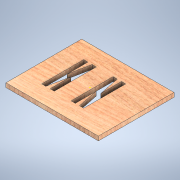
# Autodesk Inventor part: Parte A-B
Saved by Autodesk Inventor 2022 (Build 260153000, 153)
## iProperties
Created: 2023-02-12
Part Number: Parte A-B
Material: Madera (abedul)
Document SubType Name: Modeling
Designer: USUARIO
Density: 0.55 g/cm^3
Appearance: Abedul - Natural pulido
Author: USUARIO
Autodesk Inventor part; units mm, degrees
ref_plane "YZ Plane" through (0, 0, 0) normal (1, 0, 0) x (0, 1, 0)
ref_plane "XZ Plane" through (0, 0, 0) normal (0, 1, 0) x (-1, 0, 0)
ref_plane "XY Plane" through (0, 0, 0) normal (0, 0, 1) x (1, 0, 0)
sketch "Boceto1" plane through (0, 0, 0) normal (0, 1, 0) x (-1, 0, 0)
  point P0 (0, 0)
sketch "Boceto2" plane through (0, 0, 0) normal (0, 1, 0) x (-1, 0, 0)
  line L0 (110, 90) -> (-110, 90)
  line L1 (-110, 90) -> (-110, -90)
  line L2 (-110, -90) -> (110, -90)
  line L3 (110, -90) -> (110, 90)
  line L4 (110, 90) -> (-110, -90) construction
  line L5 (-110, 90) -> (110, -90) construction
  point P0 (0, 0)
  dimension "d0" = 220
  dimension "d1" = 180
  constraints: 12 end point, 2 midpoint, 2 parallel, 1 horizontal, 1 perpendicular
  measures "d0" distance of L2.end L1.end
  measures "d1" distance of L1.end L0.end
extrude "Extrusión1" add sketch "Boceto2" along normal blind 10
sketch "Boceto3" plane through (0, 10, 0) normal (0, 1, 0) x (1, 0, 0)
  point P0 (0, 0)
sketch "Boceto4" plane through (0, 10, 0) normal (0, 1, 0) x (1, 0, 0)
  line L0 (-110, 90) -> (-110, -90) projected
  line L1 (-110, 0) -> (-60, 0)
  line L2 (-110, 0) -> (-60, 0) construction
  line L3 (-65, -50) -> (-55, -50)
  line L4 (-55, -50) -> (-55, 50)
  line L5 (-55, 50) -> (-65, 50)
  line L6 (-65, 50) -> (-65, -50)
  line L7 (-65, -50) -> (-55, 50) construction
  line L8 (-55, -50) -> (-65, 50) construction
  line L9 (-55, -50) -> (-64.802, -48.0198)
  line L10 (-55, -50) -> (-45, -50) construction
  line L11 (-64.802, -48.0198) -> (-45, 50)
  line L12 (-55, -50) -> (-35.198, 48.0198)
  line L13 (-35.198, 48.0198) -> (-45, 50)
  line L14 (-55, 50) -> (-49.1181, 50)
  line L15 (-45, 50) -> (-35, 50)
  line L16 (-35, 50) -> (-35, -50)
  line L17 (-35, -50) -> (-45, -50)
  line L18 (-45, -50) -> (-45, 50)
  line L19 (-35, 0) -> (-15, 0)
  line L20 (-15, 0) -> (-15, -90)
  line L21 (35, -50) -> (25, -50)
  line L22 (25, -50) -> (25, 50)
  line L23 (25, 50) -> (35, 50)
  line L24 (35, 50) -> (35, -50)
  line L25 (35, -50) -> (25, 50) construction
  line L26 (25, -50) -> (35, 50) construction
  line L27 (25, -50) -> (34.802, -48.0198)
  line L28 (25, -50) -> (15, -50) construction
  line L29 (34.802, -48.0198) -> (15, 50)
  line L30 (25, -50) -> (5.198, 48.0198)
  line L31 (5.198, 48.0198) -> (15, 50)
  line L32 (25, 50) -> (19.1181, 50)
  line L33 (15, 50) -> (5, 50)
  line L34 (5, 50) -> (5, -50)
  line L35 (5, -50) -> (15, -50)
  line L36 (15, -50) -> (15, 50)
  line L37 (0, 0) -> (20, 0)
  line L38 (-110, -90) -> (110, -90) projected
  point P0 (30, 0)
  point P1 (30, 0)
  point P2 (5, 0)
  point P3 (15, -0.5)
  point P4 (25, 0.5)
  point P5 (-30, 50)
  point P6 (-55, 0.5)
  point P7 (-45, -0.5)
  point P8 (-70, 50)
  point P9 (-0.8819, 50)
  point P10 (15.101, 0)
  point P11 (15, 0)
  point P12 (14.899, 0)
  point P13 (15, 0)
  dimension "d4" = 50
  dimension "d5" = 0
  dimension "d6" = 10
  dimension "d7" = 100
  dimension "d8" = 10
  dimension "d10" = 100
  dimension "d11" = 100
  dimension "d12" = 10
  dimension "d13" = 100
  dimension "d14" = 20
  dimension "d15" = 20
  constraints: 74 end point, 15 symmetric about line, 8 horizontal, 6 midpoint, 5 perpendicular, 4 parallel, 2 equal length, 2 point on line
  measures "d4" distance of L1.start L1.end
  measures "d5" distance between parallel lines of L1 L2
  measures "d6" distance of L5.end L4.end
  measures "d7" distance of L4.end L3.end
  measures "d8" distance of L3.end L9.end
  measures "d10" distance of L9.end L11.end
  measures "d11" distance of L3.end L12.end
  measures "d12" distance of L16.end L17.end
  measures "d13" distance of L15.end L16.end
  measures "d14" distance of L19.start L19.end
  measures "d15" distance of L37.start L37.end
extrude "Extrusión2" cut sketch "Boceto4" against normal up to surface (10 mm away) contours L6 L5 L4 L11 L9 L3 | L9 L11 L4 | L4 L11 L18 L12 | L16 L17 L18 L12 L13 L15 | L18 L13 L12 | L21 L27 L29 L22 L23 L24 | L30 L36 L29 L22 | L22 L29 L27 | L36 L35 L34 L37 L30 | L36 L37 L30 L31 | L31 L30 L37 L34 L33
equation "\"d0\" = alto_t"
equation "\"d1\" = ancho_t"
equation "\"d2\" = grueso_t"
equation "\"d4\" = d_ranura"
equation "\"d6\" = alto_p"
equation "\"d7\" = ancho_p"
equation "\"d8\" = alto_p"
equation "\"d10\" = ancho_p"
equation "\"d11\" = ancho_p"
equation "\"d12\" = alto_p"
equation "\"d13\" = ancho_p"
equation "\"d14\" = d_sim"
equation "\"d15\" = d_sim"
equation "\"ancho_t\" = 180"
equation "\"alto_t\" = 220"
equation "\"grueso_t\" = 10"
equation "\"d_ranura\" = 50"
equation "\"ancho_p\" = 100"
equation "\"alto_p\" = 10"
equation "\"angulo_p\" = 165deg"
equation "\"d_sim\" = 20"
